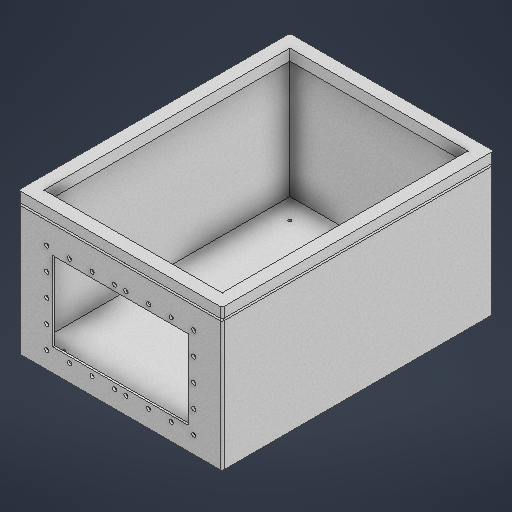
# Autodesk Inventor part: EMI-Filter-Box
Saved by Autodesk Inventor 2026.2 (Build 302298010, 298A)
## iProperties
Created: 2026-07-30
Part Number: EMI-Filter-Box
Material: Generic
Document SubType Name: Modeling
Designer: sonata
Density: 1 g/cm^3
Appearance: Default
Author: sonata
Autodesk Inventor part; units mm, degrees
ref_plane "YZ Plane" through (0, 0, 0) normal (1, 0, 0) x (0, 1, 0)
ref_plane "XZ Plane" through (0, 0, 0) normal (0, 1, 0) x (-1, 0, 0)
ref_plane "XY Plane" through (0, 0, 0) normal (0, 0, 1) x (1, 0, 0)
sketch "Sketch1" plane through (0, 0, 0) normal (0, 1, 0) x (-1, 0, 0)
  line L0 (2.286, 0) -> (226.314, 0)
  line L1 (228.6, -2.286) -> (228.6, -302.514)
  line L2 (226.314, -304.8) -> (2.286, -304.8)
  line L3 (0, -302.514) -> (0, -2.286)
  arc A0 (228.6, -2.286) -> (226.314, 0) centre (226.314, -2.286) ccw
  arc A1 (226.314, -304.8) -> (228.6, -302.514) centre (226.314, -302.514) ccw
  arc A2 (0, -302.514) -> (2.286, -304.8) centre (2.286, -302.514) ccw
  arc A3 (2.286, 0) -> (0, -2.286) centre (2.286, -2.286) ccw
  point P0 (0, 0)
  point P1 (228.6, -304.8)
  point P2 (228.6, 0)
  dimension "d0" = 304.8
  dimension "d1" = 228.6
  dimension "d2" = 2.286
  dimension "d3" = 2.286
  constraints: 8 end point, 8 point on circle, 8 tangent, 6 point on line, 4 centre point, 2 equal radius, 2 parallel, 1 horizontal, 1 perpendicular
  measures "d0" distance of point (228.6, 0) point (228.6, -304.8)
  measures "d1" distance of point (0, 0) point (228.6, 0)
  measures "d2" radius of A0
  measures "d3" radius of A1
extrude "Extrusion1" add sketch "Sketch1" along normal blind 146.05
sketch "Sketch3" plane through (0, 146.05, 0) normal (0, 1, 0) x (1, 0, 0)
  line L0 (-226.314, 2.286) -> (-2.286, 2.286)
  line L1 (-2.286, 2.286) -> (-2.286, 302.514)
  line L2 (-2.286, 302.514) -> (-226.314, 302.514)
  line L3 (-226.314, 302.514) -> (-226.314, 2.286)
  line L4 (-226.314, 0) -> (-2.286, 0) projected
  line L5 (-228.6, 302.514) -> (-228.6, 2.286) projected
  line L6 (-2.286, 304.8) -> (-226.314, 304.8) projected
  line L7 (0, 2.286) -> (0, 302.514) projected
  point P0 (0, 0)
  dimension "d6" = 2.286
  dimension "d7" = 2.286
  dimension "d8" = 2.286
  dimension "d9" = 2.286
  constraints: 8 end point, 2 parallel, 1 horizontal, 1 perpendicular
  measures "d6" distance between parallel lines of L4 L0
  measures "d7" distance between parallel lines of L5 L3
  measures "d8" distance between parallel lines of L6 L2
  measures "d9" distance between parallel lines of L7 L1
extrude "Extrusion2" cut sketch "Sketch3" against normal blind 143.764
sketch "Sketch4" plane through (-226.314, 0, 0) normal (0, 0, 1) x (1, 0, 0)
  line L0 (35.814, 114.3) -> (188.214, 114.3)
  line L1 (188.214, 114.3) -> (188.214, 25.4)
  line L2 (188.214, 25.4) -> (35.814, 25.4)
  line L3 (35.814, 25.4) -> (35.814, 114.3)
  line L4 (226.314, 0) -> (226.314, 146.05) projected
  line L5 (0, 0) -> (224.028, 0) projected
  dimension "d12" = 88.9
  dimension "d13" = 152.4
  dimension "d14" = 38.1
  dimension "d15" = 25.4
  constraints: 8 end point, 2 parallel, 1 horizontal, 1 perpendicular
  measures "d12" distance of L0.end L1.end
  measures "d13" distance of L1.end L2.end
  measures "d14" distance between parallel lines of L4 L1
  measures "d15" distance between parallel lines of L5 L2
extrude "Extrusion3" cut sketch "Sketch4" against normal up to next
sketch "Sketch5" plane through (0, 146.05, 0) normal (0, 1, 0) x (1, 0, 0)
  line L0 (-2.286, 0) -> (-226.314, 0)
  line L1 (-228.6, 2.286) -> (-228.6, 302.514)
  line L2 (-226.314, 304.8) -> (-2.286, 304.8)
  line L3 (0, 302.514) -> (0, 2.286)
  arc A0 (-226.314, 304.8) -> (-228.6, 302.514) centre (-226.314, 302.514) ccw
  arc A1 (0, 302.514) -> (-2.286, 304.8) centre (-2.286, 302.514) ccw
  arc A2 (-2.286, 0) -> (0, 2.286) centre (-2.286, 2.286) ccw
  arc A3 (-228.6, 2.286) -> (-226.314, 0) centre (-226.314, 2.286) ccw
  point P0 (0, 0)
  point P1 (-228.6, 304.8)
  point P2 (-228.6, 0)
  point P3 (0, 304.8)
  dimension "d18" = 228.6
  dimension "d19" = 304.8
  dimension "d20" = 2.286
  constraints: 8 end point, 8 point on circle, 8 point on line, 8 tangent, 4 centre point, 3 equal radius, 2 parallel, 1 horizontal, 1 perpendicular
  measures "d18" distance of point (-228.6, 304.8) point (0, 304.8)
  measures "d19" distance of point (-228.6, 0) point (-228.6, 304.8)
  measures "d20" radius of A0
fillet "Fillet1" radius 1.27 8 edges at (-0.6696, 146.05, -304.1304) (-114.3, 146.05, -304.8) (-227.9304, 146.05, -304.1304) (-228.6, 146.05, -152.4) (-227.9304, 146.05, -0.6696) (-114.3, 146.05, 0) (-0.6696, 146.05, -0.6696) (0, 146.05, -152.4)
extrude "Extrusion5" add sketch "Sketch5" along normal blind 12.7
fillet "Fillet2" radius 1.27 8 edges at (-0.6696, 146.05, -0.6696) (0, 146.05, -152.4) (-0.6696, 146.05, -304.1304) (-114.3, 146.05, -304.8) (-227.9304, 146.05, -304.1304) (-228.6, 146.05, -152.4) (-227.9304, 146.05, -0.6696) (-114.3, 146.05, 0)
sketch "Sketch6" plane through (0, 158.75, 0) normal (0, 1, 0) x (1, 0, 0)
  line L0 (-214.2998, 290.4998) -> (-14.2875, 290.4998)
  line L1 (-14.2875, 290.4998) -> (-14.2875, 14.3002)
  line L2 (-14.2875, 14.3002) -> (-214.2998, 14.3002)
  line L3 (-214.2998, 14.3002) -> (-214.2998, 290.4998)
  line L4 (0, 2.286) -> (0, 302.514) projected
  line L5 (-226.314, 0) -> (-2.286, 0) projected
  line L6 (-228.6, 302.514) -> (-228.6, 2.286) projected
  line L7 (-2.286, 304.8) -> (-226.314, 304.8) projected
  point P0 (0, 0)
  dimension "d27" = 14.2875
  dimension "d28" = 14.3002
  dimension "d29" = 14.3002
  dimension "d30" = 14.3002
  constraints: 8 end point, 2 parallel, 1 horizontal, 1 perpendicular
  measures "d27" distance between parallel lines of L4 L1
  measures "d28" distance between parallel lines of L5 L2
  measures "d29" distance between parallel lines of L6 L3
  measures "d30" distance between parallel lines of L7 L0
extrude "Extrusion6" cut sketch "Sketch6" against normal blind 12.7
sketch "Sketch7" plane through (-226.314, 0, 0) normal (0, 0, 1) x (1, 0, 0)
  line L0 (35.814, 114.3) -> (188.214, 114.3) projected
  line L1 (188.214, 114.3) -> (188.214, 25.4) projected
  line L2 (35.814, 25.4) -> (35.814, 114.3) projected
  line L3 (188.214, 25.4) -> (35.814, 25.4) projected
  point P0 (226.314, 0)
  point P1 (105.664, 120.65)
  point P2 (118.364, 120.65)
  point P3 (143.764, 120.65)
  point P4 (169.164, 120.65)
  point P5 (194.564, 120.65)
  point P6 (80.264, 120.65)
  point P7 (54.864, 120.65)
  point P8 (29.464, 120.65)
  point P9 (29.464, 95.25)
  point P10 (29.464, 69.85)
  point P11 (29.464, 44.45)
  point P12 (29.464, 19.05)
  point P13 (54.864, 19.05)
  point P14 (80.264, 19.05)
  point P15 (105.664, 19.05)
  point P16 (118.364, 19.05)
  point P17 (143.764, 19.05)
  point P18 (169.164, 19.05)
  point P19 (194.564, 19.05)
  point P20 (194.564, 44.45)
  point P21 (194.564, 69.85)
  point P22 (194.564, 95.25)
  dimension "d33" = 6.35
  dimension "d34" = 25.4
  dimension "d35" = 25.4
  dimension "d36" = 25.4
  dimension "d37" = 6.35
  dimension "d38" = 6.35
  dimension "d39" = 25.4
  dimension "d40" = 25.4
  dimension "d41" = 25.4
  dimension "d42" = 6.35
  dimension "d43" = 25.4
  dimension "d44" = 25.4
  dimension "d45" = 25.4
  dimension "d46" = 25.4
  constraints: 17 horizontal alignment, 13 vertical alignment
  measures "d33" distance from line of point (143.764, 120.65) L0
  measures "d34" distance of point (143.764, 120.65) point (118.364, 120.65)
  measures "d35" distance of point (169.164, 120.65) point (143.764, 120.65)
  measures "d36" distance of point (194.564, 120.65) point (169.164, 120.65)
  measures "d37" distance from line of point (194.564, 120.65) L1
  measures "d38" distance from line of point (29.464, 120.65) L2
  measures "d39" distance of point (54.864, 120.65) point (29.464, 120.65)
  measures "d40" distance of point (80.264, 120.65) point (54.864, 120.65)
  measures "d41" distance of point (105.664, 120.65) point (80.264, 120.65)
  measures "d42" distance from line of L3 point (29.464, 19.05)
  measures "d43" distance of point (29.464, 44.45) point (29.464, 19.05)
  measures "d44" distance of point (29.464, 69.85) point (29.464, 44.45)
  measures "d45" distance of point (29.464, 95.25) point (29.464, 69.85)
  measures "d46" distance of point (29.464, 120.65) point (29.464, 95.25)
hole "Hole1" at (-120.65, 120.65, 0) at (-107.95, 120.65, 0) at (-82.55, 120.65, 0) at (-57.15, 120.65, 0) at (-31.75, 120.65, 0) at (-146.05, 120.65, 0) at (-171.45, 120.65, 0) at (-196.85, 120.65, 0) at (-196.85, 95.25, 0) at (-196.85, 69.85, 0) at (-196.85, 44.45, 0) at (-196.85, 19.05, 0) at (-171.45, 19.05, 0) at (-146.05, 19.05, 0) at (-120.65, 19.05, 0) at (-107.95, 19.05, 0) at (-82.55, 19.05, 0) at (-57.15, 19.05, 0) at (-31.75, 19.05, 0) at (-31.75, 44.45, 0) at (-31.75, 69.85, 0) at (-31.75, 95.25, 0) direction (0, 0, -1) diameter 4.7498 depth 2.286
sketch "Sketch8" plane through (0, 0, 0) normal (0, -1, 0) x (1, 0, 0)
  line L0 (-226.314, 0) -> (-2.286, 0) projected
  line L1 (-228.6, -302.514) -> (-228.6, -2.286) projected
  line L2 (0, -2.286) -> (0, -302.514) projected
  line L3 (-2.286, -304.8) -> (-226.314, -304.8) projected
  point P0 (0, 0)
  point P1 (-203.2, -25.4)
  point P2 (-25.4, -25.4)
  point P3 (-25.4, -279.4)
  point P4 (-203.2, -279.4)
  dimension "d54" = 25.4
  dimension "d55" = 25.4
  dimension "d56" = 25.4
  dimension "d57" = 25.4
  dimension "d58" = 25.4
  dimension "d59" = 25.4
  constraints: 2 vertical alignment
  measures "d54" distance from line of L0 point (-203.2, -25.4)
  measures "d55" distance from line of L1 point (-203.2, -25.4)
  measures "d56" distance from line of L0 point (-25.4, -25.4)
  measures "d57" distance from line of L2 point (-25.4, -25.4)
  measures "d58" distance from line of point (-203.2, -279.4) L3
  measures "d59" distance from line of point (-25.4, -279.4) L3
hole "Hole2" at (-203.2, 0, -25.4) at (-25.4, 0, -25.4) at (-25.4, 0, -279.4) at (-203.2, 0, -279.4) direction (0, 1, 0) diameter 3.302 depth 2.286 thread size "8-32 UNC" class "2B" standard "ANSI Unified Screw Threads"
sketch "Sketch9" plane through (0, 0, 0) normal (0, -1, 0) x (1, 0, 0)
  circle A0 centre (-203.2, -25.4) radius 1.651 projected
  circle A1 centre (-203.2, -25.4) radius 11.43
  circle A2 centre (-25.4, -25.4) radius 1.651 projected
  circle A3 centre (-25.4, -25.4) radius 11.43
  circle A4 centre (-203.2, -279.4) radius 1.651 projected
  circle A5 centre (-203.2, -279.4) radius 11.43
  circle A6 centre (-25.4, -279.4) radius 1.651 projected
  circle A7 centre (-25.4, -279.4) radius 11.43
  point P0 (0, 0)
  dimension "d67" = 22.86
  dimension "d68" = 22.86
  dimension "d69" = 22.86
  dimension "d70" = 22.86
  constraints: 4 centre point, 4 coincident
  measures "d67" diameter of A5
  measures "d68" diameter of A1
  measures "d69" diameter of A3
  measures "d70" diameter of A7
extrude "Extrusion7" add sketch "Sketch9" along normal blind 7.62 contours A0 | A1 | A3 | A4 | A5 | A7
fillet "Fillet3" radius 5.08 4 edges at (-214.63, -7.62, -25.4) (-36.83, -7.62, -25.4) (-36.83, -7.62, -279.4) (-214.63, -7.62, -279.4)
sketch "Sketch12" plane through (-203.2, -7.62, -25.4) normal (0, -1, 0) x (1, 0, 0)
  circle A0 centre (0, 0) radius 1.651 projected
  circle A1 centre (0, 0) radius 6.35
  circle A2 centre (177.8, 0) radius 1.651 projected
  circle A3 centre (177.8, 0) radius 6.35
  circle A4 centre (0, -254) radius 1.651 projected
  circle A5 centre (0, -254) radius 6.35
  circle A6 centre (177.8, -254) radius 1.651 projected
  circle A7 centre (177.8, -254) radius 6.35
  point P0 (203.2, 25.4)
  dimension "d74" = 12.7
  dimension "d75" = 12.7
  dimension "d76" = 12.7
  dimension "d77" = 12.7
  constraints: 4 centre point, 4 coincident
  measures "d74" diameter of A1
  measures "d75" diameter of A3
  measures "d76" diameter of A5
  measures "d77" diameter of A7
extrude "Extrusion8" cut sketch "Sketch12" against normal blind 7.62 contours A0 | A1 | A2 | A3 | A4 | A5 | A6 | A7
body "Solid1"
